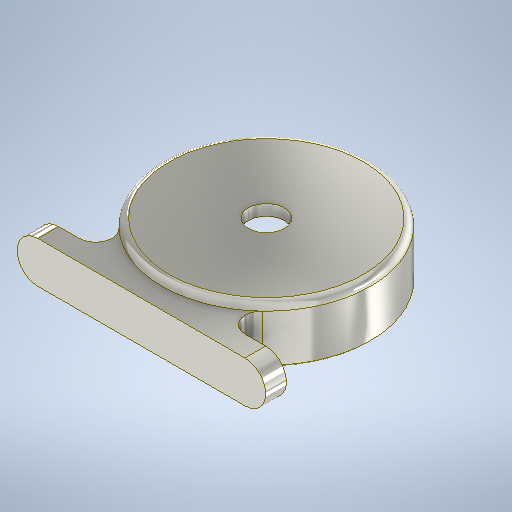
# Autodesk Inventor part: 101 part 2
Saved by Autodesk Inventor 2025.1 (Build 291241000, 241)
## iProperties
Created: 2024-09-02
Part Number: 101 part 2
Material: Silver
Document SubType Name: Modeling
Designer: ffogue
Density: 10.49 g/cm^3
Appearance: Silver
Author: ffogue
Autodesk Inventor part; units mm, degrees
ref_plane "YZ Plane" through (0, 0, 0) normal (1, 0, 0) x (0, 1, 0)
ref_plane "XZ Plane" through (0, 0, 0) normal (0, 1, 0) x (-1, 0, 0)
ref_plane "XY Plane" through (0, 0, 0) normal (0, 0, 1) x (1, 0, 0)
sketch "Sketch1" plane through (0, 0, 0) normal (0, 0, 1) x (1, 0, 0)
  line L0 (-90, 0) -> (90, 0)
  line L1 (90, 0) -> (90, 15)
  line L2 (90, 15) -> (60.1997, 15)
  arc A0 (51.9437, 35.7086) -> (60.1997, 15) centre (60.1997, 27) ccw
  circle A1 centre (0, 90.5) radius 75.5
  line L3 (-90, 0) -> (-90, 15)
  line L4 (-90, 15) -> (-60.1997, 15)
  arc A2 (-60.1997, 15) -> (-51.9437, 35.7086) centre (-60.1997, 27) ccw
  point P0 (0, 0)
  point P1 (0, 0)
  dimension "d3" = 151
  dimension "d0" = 15
  dimension "d1" = 12
  dimension "d2" = 90.5
  dimension "d4" = 180
  constraints: 10 end point, 4 point on circle, 3 horizontal alignment, 3 perpendicular, 2 centre point, 2 coincident, 2 tangent, 1 horizontal, 1 midpoint, 1 vertical, 1 vertical alignment, 5 other
  measures "d0" distance of L0.end L1.end
  measures "d1" radius of A0
  measures "d2" distance from line of L0 point (0, 90.5)
  measures "d4" distance of L0.start L0.end
extrude "Extrusion1" add sketch "Sketch1" along normal mid plane 30 contours L3 L4 A2 A1 A0 L2 L1 L0
extrude "Extrusion2" add sketch "Sketch1" along normal mid plane 40 contours A1
sketch "Sketch2" plane through (0, 90.5, -20) normal (0, 0, -1) x (-1, 0, 0)
  circle A0 centre (0, 0) radius 67.5
  point P0 (0, -90.5)
  dimension "d9" = 135
  constraints: 1 centre point, 1 vertical alignment
  measures "d9" diameter of A0
extrude "Extrusion3" cut sketch "Sketch2" against normal blind 32
fillet "Fillet1" radius 2 1 edges at (67.5, 90.5, 12)
sketch "Sketch3" plane through (0, 90.5, 12) normal (0, 0, -1) x (-1, 0, 0)
  line L0 (-90, -90.5) -> (90, -90.5) projected
  point P0 (0, -90.5)
  point P1 (0, 0)
  point P2 (0, -90.5)
  dimension "d20" = 90.5
  constraints: 1 midpoint, 1 vertical alignment
  measures "d20" distance from line of L0 point (0, 0)
hole "Hole1" at (0, 90.5, 12) direction (0, 0, 1) diameter 26 end through all
fillet "Fillet3" radius 15 4 edges at (-90, 7.5, -15) (-90, 7.5, 15) (90, 7.5, -15) (90, 7.5, 15)
fillet "Fillet4" radius 5 1 edges at (-75.5, 90.5, 20)
fillet "Fillet5" radius 1 1 edges at (-75.5, 90.5, -20)
sketch "Sketch6" plane through (0, 90.5, -20) normal (0, 0, -1) x (-1, 0, 0)
  circle A0 centre (0, 0) radius 71.5 construction
  circle A1 centre (0, 0) radius 13 projected
  point P0 (0, -90.5)
  point P1 (0, 71.5)
  dimension "d43" = 143
  constraints: 3 vertical alignment, 2 other
hole "Hole4" at (0, 162, -20) direction (0, 0, 1) diameter 4.134 depth 15 thread size "M5x0.8" class "6H" standard "ISO Metric profile"
pattern_circular "Circular Pattern2" count 12 over 360 about axis through (0, 90.5, -20) along (0, 0, 1) of "Hole4"
body "Solid1"
